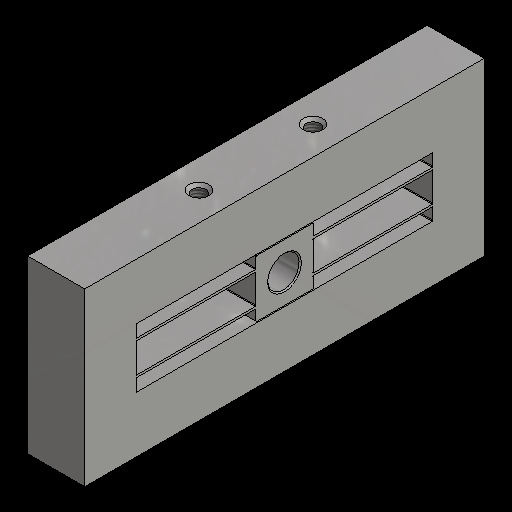
# Autodesk Inventor part: Part1
Saved by Autodesk Inventor 2025.2 (Build 292293000, 293)
## iProperties
Created: 2025-04-14
Part Number: Part1
Material: Steel ASTM A36
Document SubType Name: Modeling
Designer: Kacper Mik
Mass: 129.442 g
Surface Area: 89.2321 cm^2
Volume: 16.5951 cm^3
Density: 7.8 g/cm^3
Appearance: Steel
Author: Kacper Mik
Autodesk Inventor part; units mm, degrees
ref_plane "YZ Plane" through (0, 0, 0) normal (1, 0, 0) x (0, 1, 0)
ref_plane "XZ Plane" through (0, 0, 0) normal (0, 1, 0) x (-1, 0, 0)
ref_plane "XY Plane" through (0, 0, 0) normal (0, 0, 1) x (1, 0, 0)
sketch "Sketch1" plane through (0, 0, 0) normal (0, 1, 0) x (-1, 0, 0)
  line L0 (15, 35) -> (-15, 35)
  line L1 (-15, 35) -> (-15, -35)
  line L2 (-15, -35) -> (15, -35)
  line L3 (15, -35) -> (15, 35)
  line L4 (15, 35) -> (-15, -35) construction
  line L5 (-15, 35) -> (15, -35) construction
  point P0 (0, 0)
  dimension "d0" = 30
  dimension "d1" = 70
  constraints: 12 end point, 2 midpoint, 2 parallel, 1 horizontal, 1 perpendicular
  measures "d0" distance of L2.end L1.end
  measures "d1" distance of L1.end L0.end
extrude "gabaryty" add sketch "Sketch1" along normal blind 10
sketch "Sketch2" plane through (0, 10, 0) normal (0, 1, 0) x (1, 0, 0)
  line L0 (5.2, -26) -> (-5.2, -26)
  line L1 (-5.2, -26) -> (-5.2, 26)
  line L2 (-5.2, 26) -> (5.2, 26)
  line L3 (5.2, 26) -> (5.2, -26)
  line L4 (5.2, -26) -> (-5.2, 26) construction
  line L5 (-5.2, -26) -> (5.2, 26) construction
  point P0 (0, 0)
  dimension "d4" = 10.4
  dimension "d5" = 52
  constraints: 12 end point, 2 midpoint, 2 parallel, 1 horizontal, 1 perpendicular
  measures "d4" distance of L1.end L2.end
  measures "d5" distance of L0.end L1.end
extrude "przestrzen srodek" cut sketch "Sketch2" against normal through all
sketch "Sketch3" plane through (0, 10, 0) normal (0, 1, 0) x (1, 0, 0)
  line L0 (5, 5) -> (-5, 5)
  line L1 (-5, 5) -> (-5, -5)
  line L2 (-5, -5) -> (5, -5)
  line L3 (5, -5) -> (5, 5)
  line L4 (5, 5) -> (-5, -5) construction
  line L5 (-5, 5) -> (5, -5) construction
  point P0 (0, 0)
  dimension "d8" = 10
  dimension "d9" = 10
  constraints: 12 end point, 2 midpoint, 2 parallel, 1 horizontal, 1 perpendicular
  measures "d8" distance of L2.end L1.end
  measures "d9" distance of L1.end L0.end
extrude "bloczek srodek" add sketch "Sketch3" against normal blind 10
sketch "Sketch4" plane through (0, 10, 0) normal (0, 1, 0) x (1, 0, 0)
  line L0 (-5, 5) -> (-5, -5) construction
  line L1 (-5, -5) -> (5, -5) construction
  line L2 (5, -5) -> (5, 5) construction
  line L3 (5, 5) -> (-5, 5) construction
  line L4 (-5.2, -26) -> (-5.2, 26) construction
  line L5 (-5.2, 26) -> (5.2, 26) construction
  line L6 (5.2, 26) -> (5.2, -26) construction
  line L7 (5.2, -26) -> (-5.2, -26) construction
  line L8 (15, -35) -> (15, 35) construction
  line L9 (15, 35) -> (-15, 35) construction
  line L10 (-15, 35) -> (-15, -35) construction
  line L11 (-15, -35) -> (15, -35) construction
  line L12 (-5.2, -26) -> (5.2, -26) projected
  line L13 (-3, -5) -> (-2.6, -5)
  line L14 (-2.6, -5) -> (-2.6, -26)
  line L15 (-2.6, -26) -> (-3, -26)
  line L16 (-3, -26) -> (-3, -5)
  line L17 (3, -5) -> (2.6, -5)
  line L18 (2.6, -5) -> (2.6, -26)
  line L19 (2.6, -26) -> (3, -26)
  line L20 (3, -26) -> (3, -5)
  line L21 (3, 5) -> (2.6, 5)
  line L22 (2.6, 5) -> (2.6, 26)
  line L23 (2.6, 26) -> (3, 26)
  line L24 (3, 26) -> (3, 5)
  line L25 (-5, 5) -> (5, 5) projected
  line L26 (-3, 5) -> (-2.6, 5)
  line L27 (-2.6, 5) -> (-2.6, 26)
  line L28 (-2.6, 26) -> (-3, 26)
  line L29 (-3, 26) -> (-3, 5)
  point P0 (0, 0)
  point P1 (-2.6, 5)
  dimension "d12" = 0.4
  dimension "d13" = 2
  dimension "d14" = 0.4
  dimension "d15" = 2
  dimension "d16" = 0.4
  dimension "d17" = 2
  dimension "d18" = 0.4
  dimension "d19" = 2
  constraints: 32 end point, 8 parallel, 8 point on line, 4 horizontal, 4 perpendicular
  measures "d12" distance of L14.end L15.end
  measures "d13" distance from line of L0 L13.start
  measures "d14" distance of L19.end L18.end
  measures "d15" distance between parallel lines of L2 L20
  measures "d16" distance between parallel lines of L27 L29
  measures "d17" distance between parallel lines of L0 L29
  measures "d18" distance between parallel lines of L24 L22
  measures "d19" distance between parallel lines of L2 L24
extrude "Belki" add sketch "Sketch4" against normal blind 10
sketch "Sketch5" plane through (0, 10, 0) normal (0, 1, 0) x (1, 0, 0)
  point P0 (0, 0)
  point P1 (0, 0)
  constraints: 1 coincident
hole "srodek" at (0, 10, 0) direction (0, -1, 0) diameter 5.5 end through all clearance for "Slotted Cheese Head Screw ISO 1207" size "M5" standard "ISO"
sketch "Sketch6" plane through (-15, 0, -35) normal (-1, 0, 0) x (0, 0, 1)
  line L0 (0, 0) -> (70, 0) construction
  line L1 (70, 0) -> (70, 10) construction
  line L2 (0, 10) -> (70, 10) construction
  line L3 (0, 0) -> (0, 10) construction
  line L4 (35, 0) -> (35, 10) construction
  point P0 (45, 5)
  point P1 (25, 5)
  dimension "d29" = 10
  dimension "d30" = 10
  dimension "d31" = 5
  dimension "d32" = 5
  constraints: 2 end point, 1 midpoint
  measures "d29" distance from line of L4 point (45, 5)
  measures "d30" distance from line of point (25, 5) L4
  measures "d31" distance from line of L2 point (45, 5)
  measures "d32" distance from line of L2 point (25, 5)
hole "mocowanie gora" at (-15, 5, 10) at (-15, 5, -10) direction (1, 0, 0) diameter 2.459 depth 9.8 thread size "M3x0.5" class "6H" standard "ISO Metric profile"
chamfer "Chamfer1" distance 0.5 angle 45 2 edges at (-15, 5, -11.2295) (-15, 5, 8.7705)
fillet "zaokraglenie lasera" radius 0.1 24 edges at (-3, 5, 5) (-2.6, 5, 5) (-3, 5, 26) (-2.6, 5, 26) (2.6, 5, 26) (2.6, 5, 5) (3, 5, 5) (3, 5, 26) (3, 5, -5) (2.6, 5, -5) (-2.6, 5, -5) (-3, 5, -5) (-3, 5, -26) (2.6, 5, -26) (-2.6, 5, -26) (3, 5, -26) (-5.2, 5, 26) (-5.2, 5, -26) (5.2, 5, -26) (5.2, 5, 26) (-5, 5, 5) (-5, 5, -5) (5, 5, -5) (5, 5, 5)
chamfer "Chamfer2" distance 0.2 angle 45 1 edges at (0, 10, -2.75)
equation "\"d14\" = d12"
equation "\"d15\" = d13"
equation "\"d16\" = d12"
equation "\"d17\" = d13"
equation "\"d18\" = d12"
equation "\"d19\" = d13"
equation "\"d30\" = d29"
equation "\"d32\" = d31"
body "Solid1"
